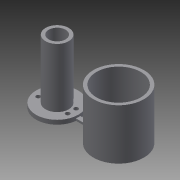
# Autodesk Inventor part: Bobbin01
Saved by Autodesk Inventor 2015 (Build 190159000, 159)
## iProperties
Created: 2016-06-12
Part Number: Bobbin01
Material: Generic
Document SubType Name: Modeling
Designer: Alex
Density: 1 g/cm^3
Appearance: Default
Author: Alex
Autodesk Inventor part; units mm, degrees
ref_plane "YZ Plane" through (0, 0, 0) normal (1, 0, 0) x (0, 1, 0)
ref_plane "XZ Plane" through (0, 0, 0) normal (0, 1, 0) x (-1, 0, 0)
ref_plane "XY Plane" through (0, 0, 0) normal (0, 0, 1) x (1, 0, 0)
sketch "Sketch1" plane through (0, 0, 0) normal (0, 0, 1) x (1, 0, 0)
  circle A0 centre (0, 0) radius 10
  dimension "d0" = 20
  constraints: 1 centre point, 1 coincident
  measures "d0" diameter of A0
extrude "Extrusion1" add sketch "Sketch1" along normal blind 2
sketch "Sketch2" plane through (0, 0, 0) normal (0, 0, -1) x (-1, 0, 0)
  circle A0 centre (0, 0) radius 5.5
  circle A1 centre (0, 0) radius 3.55
  dimension "d3" = 11
  dimension "d6" = 7.1
  constraints: 2 centre point, 1 coincident
  measures "d3" diameter of A0
  measures "d6" diameter of A1
extrude "Extrusion2" add sketch "Sketch2" against normal blind 30 contours A0 | A1
sketch "Sketch3" plane through (0, 0, 0) normal (0, 0, -1) x (-1, 0, 0)
  point P0 (0, 0)
sketch "Sketch4" plane through (0, 0, 0) normal (0, 0, -1) x (-1, 0, 0)
  point P0 (0, 0)
sketch "Sketch5" plane through (0, 0, 0) normal (0, 0, -1) x (-1, 0, 0)
  circle A0 centre (0, 0) radius 4
  dimension "d7" = 8
  constraints: 1 centre point, 1 coincident
  measures "d7" diameter of A0
extrude "Extrusion3" cut sketch "Sketch5" against normal blind 30
sketch "Sketch6" plane through (0, 0, 2) normal (0, 0, 1) x (1, 0, 0)
  circle A0 centre (7, 2) radius 1
  circle A1 centre (7, -2) radius 1
  circle A2 centre (-7, 2) radius 1
  circle A3 centre (-7, -2) radius 1
  point P0 (0, 0)
  dimension "d16" = 2
  dimension "d17" = 7
  dimension "d18" = 2
  dimension "d19" = 2
  dimension "d20" = 7
  dimension "d21" = 2
  dimension "d53" = 2
  dimension "d54" = 7
  dimension "d55" = 2
  dimension "d56" = 2
  dimension "d57" = 7
  dimension "d58" = 2
  constraints: 4 centre point
  measures "d16" vertical distance of point (0, 0) A0.centre
  measures "d17" horizontal distance of point (0, 0) A0.centre
  measures "d18" diameter of A0
  measures "d19" vertical distance of point (0, 0) A1.centre
  measures "d20" horizontal distance of point (0, 0) A1.centre
  measures "d21" diameter of A1
  measures "d53" diameter of A2
  measures "d54" horizontal distance of point (0, 0) A2.centre
  measures "d55" vertical distance of point (0, 0) A2.centre
  measures "d56" vertical distance of point (0, 0) A3.centre
  measures "d57" horizontal distance of point (0, 0) A3.centre
  measures "d58" diameter of A3
extrude "Extrusion4" cut sketch "Sketch6" against normal blind 2
sketch "Sketch7" plane through (0, 0, 0) normal (0, 0, -1) x (-1, 0, 0)
  point P0 (0, 0)
sketch "Sketch8" plane through (0, 0, 0) normal (0, 0, -1) x (-1, 0, 0)
  circle A0 centre (-29.1938, 0) radius 12
  point P0 (0, 0)
  dimension "d24" = 24
  constraints: 1 centre point
  measures "d24" diameter of A0
extrude "Extrusion5" add sketch "Sketch8" against normal blind 2
sketch "Sketch9" plane through (29.1938, 0, 0) normal (0, 0, -1) x (-1, 0, 0)
  circle A0 centre (0, 0) radius 6
  point P0 (29.1938, 0)
  dimension "d27" = 12
  constraints: 1 centre point
  measures "d27" diameter of A0
extrude "Extrusion6" cut sketch "Sketch9" against normal blind 1
sketch "Sketch10" plane through (29.1938, 0, 0) normal (0, 0, -1) x (-1, 0, 0)
  point P0 (29.1938, 0)
  point P1 (0, 0)
sketch "Sketch11" plane through (29.1938, 0, 0) normal (0, 0, -1) x (-1, 0, 0)
  circle A0 centre (7.6938, 2) radius 1
  circle A1 centre (-8.3062, 2) radius 1
  circle A2 centre (-8.3062, -2) radius 1
  circle A3 centre (7.6938, -2) radius 1
  point P0 (29.1938, 0)
  dimension "d30" = 21.5
  dimension "d31" = 2
  dimension "d32" = 16
  dimension "d33" = 2
  dimension "d34" = 2
  dimension "d35" = 0
  dimension "d36" = 0
  dimension "d37" = 4
  dimension "d38" = 2
  dimension "d40" = 2
  dimension "d41" = 4
  constraints: 4 centre point
  measures "d30" horizontal distance of point (29.194, 0) A0.centre
  measures "d31" diameter of A0
  measures "d32" distance of A0.centre A1.centre
  measures "d33" diameter of A1
  measures "d34" vertical distance of point (29.194, 0) A0.centre
  measures "d35" vertical distance of A0.centre A1.centre
  measures "d36" horizontal distance of A0.centre A3.centre
  measures "d37" distance of A0.centre A3.centre
  measures "d38" diameter of A3
  measures "d40" diameter of A2
  measures "d41" distance of A1.centre A2.centre
extrude "Extrusion7" cut sketch "Sketch11" against normal blind 2
sketch "Sketch12" plane through (29.1938, 0, 2) normal (0, 0, 1) x (1, 0, 0)
  circle A0 centre (0, 0) radius 4.55
  point P0 (-29.1938, 0)
  dimension "d44" = 9.1
  constraints: 1 centre point
  measures "d44" diameter of A0
extrude "Extrusion8" cut sketch "Sketch12" against normal blind 1
sketch "Sketch13" plane through (29.1938, 0, 0) normal (0, 0, -1) x (-1, 0, 0)
  line L0 (19.6938, 1) -> (11.6938, 1)
  line L1 (11.6938, 1) -> (11.6938, -1)
  line L2 (11.6938, -1) -> (19.6938, -1)
  line L3 (19.6938, -1) -> (19.6938, 1)
  point P0 (29.1938, 0)
  dimension "d47" = 8
  dimension "d48" = 2
  dimension "d49" = 1
  dimension "d50" = 9.5
  constraints: 8 end point, 2 parallel, 1 horizontal, 1 perpendicular
  measures "d47" distance of L0.start L0.end
  measures "d48" distance of L2.end L0.start
  measures "d49" distance from line of point (29.194, 0) L0
  measures "d50" distance from line of point (29.194, 0) L3
extrude "Extrusion9" add sketch "Sketch13" against normal blind 1
sketch "Sketch14" plane through (29.1938, 0, 2) normal (0, 0, 1) x (1, 0, 0)
  point P0 (-29.1938, 0)
sketch "Sketch15" plane through (29.1938, 0, 2) normal (0, 0, 1) x (1, 0, 0)
  circle A0 centre (0, 0) radius 12
  point P0 (-29.1938, 0)
  dimension "d59" = 24
  constraints: 1 centre point
  measures "d59" diameter of A0
extrude "Extrusion10" add sketch "Sketch15" along normal blind 22
sketch "Sketch16" plane through (29.1938, 0, 24) normal (0, 0, 1) x (1, 0, 0)
  circle A0 centre (0, 0) radius 10.5
  point P0 (-29.1938, 0)
  dimension "d62" = 21
  constraints: 1 centre point
  measures "d62" diameter of A0
extrude "Extrusion11" cut sketch "Sketch16" against normal blind 23
body "Solid1"
